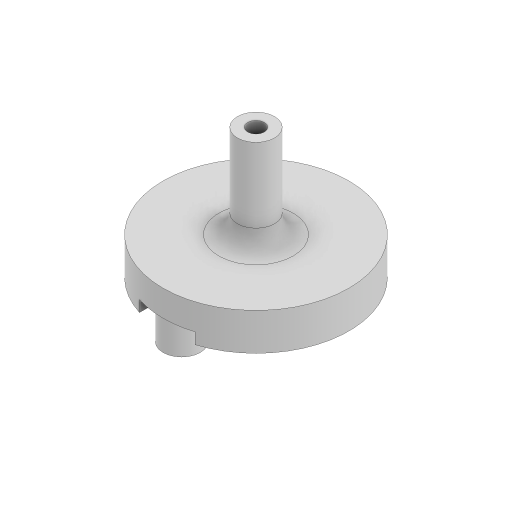
# Autodesk Inventor part: GUIA GIRATORIA
Saved by Autodesk Inventor 2024 (Build 280153000, 153)
## iProperties
Created: 2024-06-30
Part Number: GUIA GIRATORIA
Material: Generic
Document SubType Name: Modeling
Designer: Jhuliams
Density: 1 g/cm^3
Appearance: Default
Author: Jhuliams
Autodesk Inventor part; units mm, degrees
ref_plane "YZ Plane" through (0, 0, 0) normal (1, 0, 0) x (0, 1, 0)
ref_plane "XZ Plane" through (0, 0, 0) normal (0, 1, 0) x (-1, 0, 0)
ref_plane "XY Plane" through (0, 0, 0) normal (0, 0, 1) x (1, 0, 0)
sketch "Sketch1" plane through (0, 0, 0) normal (0, 1, 0) x (-1, 0, 0)
  circle A0 centre (0, 0) radius 25
  line L0 (0, 0) -> (20, 0)
  circle A1 centre (20, 0) radius 5
  line L1 (7.5, 45) -> (-7.5, 45)
  line L2 (-7.5, 45) -> (-7.5, -45)
  line L3 (-7.5, -45) -> (7.5, -45)
  line L4 (7.5, -45) -> (7.5, 45)
  line L5 (7.5, 45) -> (-7.5, -45) construction
  line L6 (-7.5, 45) -> (7.5, -45) construction
  point P0 (7.5, 23.8485)
  point P1 (-7.5, 23.8485)
  point P2 (-7.5, -23.8485)
  point P3 (7.5, -23.8485)
  dimension "d0" = 50
  dimension "d1" = 20
  dimension "d2" = 10
  dimension "d3" = 15
  dimension "d4" = 90
  constraints: 14 end point, 2 centre point, 2 coincident, 2 horizontal, 2 midpoint, 2 parallel, 1 perpendicular
  measures "d0" diameter of A0
  measures "d1" distance of L0.start L0.end
  measures "d2" diameter of A1
  measures "d3" distance of L3.end L2.end
  measures "d4" distance of L2.end L1.end
extrude "Extrusion1" add sketch "Sketch1" along normal blind 10 contours A1 L0 L4 A0 | A1 | A0 L4 L0 A1 | L4 A0 L2 | L2 A0
extrude "Extrusion2" add sketch "Sketch1" against normal blind 25 contours A1
extrude "Extrusion3" cut sketch "Sketch1" along normal blind 3 contours L4 A0 L2
sketch "Sketch2" plane through (0, 10, 0) normal (0, 1, 0) x (1, 0, 0)
  circle A0 centre (0, 0) radius 5
  circle A1 centre (0, 0) radius 2.25
  dimension "d11" = 10
  dimension "d12" = 4.5
  constraints: 2 centre point, 2 coincident
  measures "d11" diameter of A0
  measures "d12" diameter of A1
extrude "Extrusion4" add sketch "Sketch2" along normal blind 25
fillet "Fillet1" radius 5 1 edges at (-5, 10, 0)
body "Solid1"
